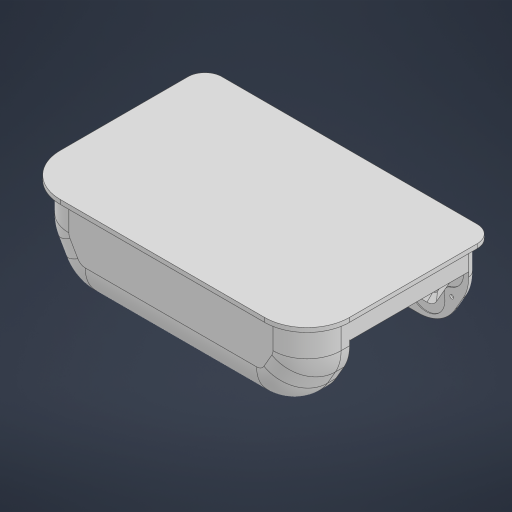
# Autodesk Inventor part: cap
Saved by Autodesk Inventor 2024 (Build 280153000, 153)
## iProperties
Created: 2024-05-06
Part Number: cap
Material: Generic
Document SubType Name: Modeling
Designer: markm
Density: 1 g/cm^3
Appearance: Default
Author: markm
Autodesk Inventor part; units mm, degrees
ref_plane "YZ Plane" through (0, 0, 0) normal (1, 0, 0) x (0, 1, 0)
ref_plane "XZ Plane" through (0, 0, 0) normal (0, 1, 0) x (-1, 0, 0)
ref_plane "XY Plane" through (0, 0, 0) normal (0, 0, 1) x (1, 0, 0)
sketch "Sketch18" plane through (0, 0, 0) normal (0, 1, 0) x (-1, 0, 0)
  line L0 (0, 55) -> (0, -55)
  line L1 (0, -55) -> (-85, -55)
  line L2 (-85, -55) -> (-85, 55)
  line L3 (0, 55) -> (-85, 55)
  point P0 (0, 0)
  point P1 (0, 0)
  dimension "d157" = 85
  dimension "d178" = 110
  constraints: 8 end point, 2 perpendicular, 1 coincident, 1 horizontal, 1 midpoint, 1 vertical
  measures "d157" distance between parallel lines of L2 L0
  measures "d178" distance between parallel lines of L3 L1
extrude "Extrusion22" add sketch "Sketch18" along normal blind 2.5
sketch "Sketch19" plane through (0, 0, 0) normal (0, -1, 0) x (1, 0, 0)
  line L0 (85, 55) -> (85, -55) projected
  line L1 (0, 55) -> (85, 55) projected
  line L2 (0, -55) -> (0, 55) projected
  line L3 (85, -55) -> (0, -55) projected
  line L4 (5, 50) -> (0, 50)
  line L5 (5, -50) -> (0, -50)
  line L6 (5, -50) -> (5, 50)
  line L7 (5, 50) -> (80, 50)
  line L8 (80, 50) -> (80, -50)
  line L9 (80, -50) -> (5, -50)
  point P0 (0, 0)
  dimension "d179" = 5
  constraints: 12 end point, 2 perpendicular, 2 point on line, 3 other
  measures "d179" distance between parallel lines of L3 L9
extrude "Extrusion23" add sketch "Sketch19" along normal blind 5 contours L4 L6 L5 L2 | L7 L8 L9 L6
sketch "Sketch20" plane through (0, -5, 0) normal (0, -1, 0) x (1, 0, 0)
  line L0 (0, 50) -> (0, -50) projected
  line L1 (80, 30) -> (0, 30)
  line L2 (80, -45) -> (0, -45)
  line L3 (80, 25) -> (0, 25)
  line L4 (0, -50) -> (80, -50) projected
  line L5 (80, -50) -> (80, 50) projected
  line L6 (80, 50) -> (0, 50) projected
  point P0 (0, 0)
  point P1 (0, 25)
  dimension "d167" = 5
  constraints: 6 end point, 3 perpendicular, 3 point on line, 1 parallel
  measures "d167" distance between parallel lines of L1 L3
extrude "Extrusion24" add sketch "Sketch20" along normal blind 45 contours L6 L5 L1 L0 | L1 L5 L3 L0 | L2 L5 L4 L0
sketch "Sketch21" plane through (0, 0, 0) normal (0, 0, 1) x (1, 0, 0)
  line L0 (0, -5) -> (80, -5)
  line L1 (0, -5) -> (0, -50)
  line L2 (80, -50) -> (0, -50)
  line L3 (80, -5) -> (80, -50)
  arc A0 (55, -47) -> (64.526279, -41.5) centre (55, -36) ccw construction
  line L4 (55, -36) -> (66, -16.947441) construction
  line L5 (0, -47) -> (55, -47) construction
  line L6 (64.526279, -41.5) -> (75.526279, -22.447441) construction
  arc A1 (75.526279, -22.447441) -> (74.887436, -10.465661) centre (66, -16.947441) ccw construction
  arc A2 (78.124356, -23.947441) -> (80, -16.947441) centre (66, -16.947441) ccw
  line L7 (78.124356, -23.947441) -> (67.124356, -43)
  arc A3 (55, -50) -> (67.124356, -43) centre (55, -36) ccw
  line L8 (55, -50) -> (0, -50)
  arc A4 (76.650635, -29.447441) -> (80, -16.947441) centre (55, -16.947441) ccw
  line L9 (76.650635, -29.447441) -> (64.78461, -50)
  arc A5 (50.350853, -50) -> (72.001488, -37.5) centre (50.350853, -25) ccw
  point P0 (0, 0)
  point P1 (55, -50)
  point P2 (50.350853, -50)
  dimension "d170" = 22
  dimension "d171" = 55
  dimension "d172" = 60
  dimension "d174" = 3
  dimension "d175" = 3
  dimension "d242" = 25
  constraints: 12 end point, 12 point on circle, 7 tangent, 6 centre point, 5 point on line, 2 equal radius, 2 parallel, 1 coincident, 3 other
  measures "d170" diameter of A0
  measures "d171" distance from line of L1 L4.start
  measures "d172" angle of L2 L4
  measures "d174" distance between parallel lines of L2 L5
  measures "d175" distance between parallel lines of L6 L7
  measures "d242" radius of A4
extrude "Extrusion25" cut sketch "Sketch21" along normal through all both and the other way through all contours L3 L2 L9 A4 | A5 A3 L2 | A3 A5 L9 L2
fillet "Fillet6" radius 20 1 edges at (80, -8.4737, 50)
fillet "Fillet6" radius 5 2 edges at (25.1754, -50, -50) (80, -8.4737, -50)
fillet "Fillet6" radius 25 1 edges at (85, 1.25, 55)
fillet "Fillet6" radius 10 1 edges at (85, 1.25, -55)
chamfer "Chamfer8" distance 5 distance2 2.5 5 edges at (74.1422, 0, 44.1422) (30, 0, 50) (80, 0, -7.5) (78.5356, 0, -48.5356) (37.5, 0, -50) measured on face at (80.5, 0, -7.5) measured on face at (37.5, 0, -50.5) measured on face at (78.8891, 0, -48.8891) measured on face at (74.4957, 0, 44.4957) measured on face at (30, 0, 50.5)
sketch "Sketch24" plane through (0, 2.5, -55) normal (-1, 0, 0) x (0, 0, 1)
  line L0 (110, -2.5) -> (105, -5) construction
  circle A0 centre (107.5, -3.75) radius 1
  point P0 (55, -2.5)
  dimension "d194" = 2
  constraints: 1 centre point, 1 midpoint
  measures "d194" diameter of A0
sketch3d "3D Sketch4"
  line L0 (0, -2.5, 50) -> (60, -2.5, 50)
  arc A0 (60, -2.5, 50) -> (80, -2.5, 30) centre (60, -2.5, 30) ccw
  line L1 (80, -2.5, 30) -> (80, -2.5, -45)
  arc A1 (80, -2.5, -45) -> (75, -2.5, -50) centre (75, -2.5, -45) ccw
  line L2 (75, -2.5, -50) -> (0, -2.5, -50)
sweep "Sweep4" cut profiles "Sketch24" path "3D Sketch4"
mirror "Mirror4" about plane through (0, 0, 0) normal (1, 0, 0)
ref_plane "Work Plane1" through (80, -16.947441, -10) normal (0, 0, 1) x (1, 0, 0)
sketch "Sketch26" plane through (80, -16.947441, -10) normal (0, 0, 1) x (1, 0, 0)
  line L0 (0, 11.947441) -> (0, 0)
  line L1 (-160, 11.947441) -> (0, 11.947441)
  line L2 (-160, 11.947441) -> (-160, 0)
  line L3 (-29.649147, -33.052559) -> (-130.350853, -33.052559)
  circle A0 centre (-25, -19.052559) radius 11
  circle A1 centre (-14.000001, 0) radius 11
  circle A2 centre (-146, 0) radius 11
  circle A3 centre (-47, -19.052559) radius 11
  circle A4 centre (-36.000001, 0) radius 11
  circle A5 centre (-69, -19.052559) radius 11
  circle A6 centre (-58.000001, 0) radius 11
  circle A7 centre (-91, -19.052559) radius 11
  circle A8 centre (-80.000001, 0) radius 11
  circle A9 centre (-113, -19.052559) radius 11
  circle A10 centre (-102.000001, 0) radius 11
  circle A11 centre (-135, -19.052559) radius 11
  circle A12 centre (-124.000001, 0) radius 11
  arc A13 (0, 0) -> (-14, 14) centre (-14, 0) ccw
  line L4 (-14, 14) -> (-146, 14)
  arc A14 (-146, 14) -> (-160, 0) centre (-146, 0) ccw
  arc A15 (-140.629165, -22.302559) -> (-135, -25.552559) centre (-135, -19.052559) ccw
  line L5 (-140.629165, -22.302559) -> (-151.629165, -3.25)
  arc A16 (-152.5, 0) -> (-151.629165, -3.25) centre (-146, 0) ccw
  line L6 (-152.5, 0) -> (-152.5, 4.447441)
  line L7 (-152.5, 4.447441) -> (-7.5, 4.447441)
  line L8 (-7.5, 4.447441) -> (-7.5, 0)
  arc A17 (-8.370835, -3.25) -> (-7.5, 0) centre (-14.000001, 0) ccw
  line L9 (-8.370835, -3.25) -> (-19.370835, -22.302559)
  arc A18 (-25, -25.552559) -> (-19.370835, -22.302559) centre (-25, -19.052559) ccw
  line L10 (-25, -25.552559) -> (-135, -25.552559)
  arc A19 (-146, 6.5) -> (-152.5, 0) centre (-146, 0) ccw
  line L11 (-146, 6.5) -> (-14, 6.5)
  arc A20 (-7.5, 0) -> (-14, 6.5) centre (-14, 0) ccw
  arc A21 (-3.349365, -12.5) -> (0, 0) centre (-25, 0) ccw
  arc A22 (-160, 0) -> (-156.650635, -12.5) centre (-135, 0) ccw
  line L12 (-152.001488, -20.552559) -> (-156.650635, -12.5)
  line L13 (-7.998512, -20.552559) -> (-3.349365, -12.5)
  arc A23 (-152.001488, -20.552559) -> (-130.350853, -33.052559) centre (-130.350853, -8.052559) ccw
  arc A24 (-29.649147, -33.052559) -> (-7.998512, -20.552559) centre (-29.649147, -8.052559) ccw
  point P0 (-80, 16.947441)
  point P1 (-153.297852, 11.947441)
  point P2 (-6.702148, 11.947441)
  point P3 (-7.5, 0)
  point P4 (-135, 0.003127)
  point P5 (-140.5, -9.526279)
  point P6 (-124, -19.052559)
  point P7 (-102, -19.052559)
  point P8 (-80, -19.052559)
  point P9 (-58, -19.052559)
  point P10 (-36, -19.052559)
  point P11 (-19.498599, -9.527088)
  point P12 (-25.000001, 0)
  point P13 (-47.000001, 0)
  point P14 (-69.000001, 0)
  point P15 (-91.000001, 0)
  point P16 (-113.000001, 0)
  dimension "d205" = 22
  dimension "d208" = 22
  dimension "d213" = 7.5
  constraints: 21 centre point, 16 end point, 16 point on circle, 3 coincident, 3 equal radius, 2 horizontal, 1 tangent, 24 other
  measures "d205" diameter of A0
  measures "d208" distance of A0.centre A3.centre
  measures "d213" distance between parallel lines of L3 L10
extrude "Extrusion28" add sketch "Sketch26" against normal up to surface (35 mm away) contours L0 A13 L1 | A14 L2 L1
extrude "Extrusion29" cut sketch "Sketch26" against normal up to surface (35 mm away) contours L1 A14 L4 A13
extrude "Extrusion31" cut sketch "Sketch26" against normal blind 35.5 contours A0 L10 A18 L9 | L9 A18 L10 A0 | A0 A4 A1 | A1 L7 A20 A17 L9 | L9 A17 L8 L7 A20 L11 A1 | A3 A4 A0 | A3 L10 | A3 L10 | A4 L7 | A3 A6 A4 | A1 L11 A20 L7 | L7 A4 L11 | A20 L7 L8 | A3 A5 A6 | A6 L7 | A5 L10 | A5 L10 | L11 A4 | A5 A8 A6 | L7 A6 L11 | A5 A7 A8 | A8 L7 | L11 A6 | A7 L10 | A7 L10 | A7 A10 A8 | L7 A8 L11 | A7 A9 A10 | A10 L7 | L11 A8 | A9 L10 | A9 L10 | A9 A12 A10 | L7 A10 L11 | A9 A11 A12 | A12 L7 | L11 A10 | A11 L10 A15 L5 | A11 L5 A15 L10 | A11 A2 A12 | L7 A12 L11 | A2 L5 A16 A19 L7 | L11 A12 | A2 L11 A19 L7 L6 A16 L5 | L7 A19 L11 A2 | A19 L6 L7
fillet "Fillet9" radius 5 13 edges at (-60.5, -26.4737, -45.25) (-44, -36, -45.25) (-22, -36, -45.25) (44, -36, -45.25) (0, -36, -45.25) (22, -36, -45.25) (-55, -16.9443, -45.25) (33, -16.9474, -45.25) (55, -16.9474, -45.25) (11, -16.9474, -45.25) (-33, -16.9474, -45.25) (-11, -16.9474, -45.25) (60.5014, -26.4745, -45.25)
extrude "Extrusion30" cut sketch "Sketch26" against normal blind 39 contours L9 A18 L10 A0 | A0 A1 L9 | L10 A3 A0 | A0 A4 A1 | A1 L7 A20 A17 L9 | A3 A4 A0 | A3 L10 | A4 L7 | A4 L7 A1 | A3 A6 A4 | L10 A5 A3 | L7 A4 L11 A1 | A1 L11 A20 L7 | L7 A4 L11 | A3 A5 A6 | A6 L7 | A6 L7 A4 | A5 L10 | L7 A6 L11 A4 | A5 A8 A6 | L7 A6 L11 | L10 A7 A5 | A5 A7 A8 | A8 L7 | A8 L7 A6 | L7 A8 L11 A6 | A7 L10 | A7 A10 A8 | L7 A8 L11 | L10 A9 A7 | A7 A9 A10 | A10 L7 | A10 L7 A8 | L7 A10 L11 A8 | A9 L10 | A9 A12 A10 | L7 A10 L11 | L10 A11 A9 | A9 A11 A12 | A12 L7 | A12 L7 A10 | L7 A12 L11 A10 | A11 L10 A15 L5 | A11 A2 A12 | L7 A12 L11 | L5 A2 A11 | A2 L5 A16 A19 L7 | A2 L7 A12 | L7 A2 L11 A12 | L7 A19 L11 A2 picked at (-24.956945, -19.127133) picked at (-44.033604, -18.431276) picked at (-72.50543, -19.057181) picked at (-94.50543, -19.057181) picked at (-116.50543, -19.057181) picked at (-135.043055, -19.127132)
chamfer "Chamfer10" distance 3.5 angle 45 10 edges at (58.25, -41.6292, -49) (0, -42.5, -49) (-58.25, -41.6292, -49) (-66.1292, -29.7237, -49) (-70.5962, -12.3512, -49) (-72.2785, -18.6298, -49) (0, -10.4474, -49) (72.2785, -18.6298, -49) (70.5962, -12.3512, -49) (66.1292, -29.7237, -49)
sketch "Sketch27" plane through (75, -16.947441, -50) normal (0, 0, -1) x (-1, 0, 0)
  line L0 (0, 14.447441) -> (150, 14.447441) construction
  line L1 (0, 0) -> (0, 14.447441) construction
  line L2 (125.350853, -28.052559) -> (24.649147, -28.052559) construction
  line L3 (150, 0) -> (150, 14.447441) construction
  arc A0 (9.300915, -16.497256) -> (5.863415, -10.543331) centre (4.437694, -15.335754) ccw construction
  arc A1 (9.300915, -16.497256) -> (27.5625, -27.040587) centre (20, -19.052559) ccw construction
  arc A2 (34.4375, -27.040587) -> (27.5625, -27.040587) centre (31, -30.671509) ccw construction
  arc A3 (34.4375, -27.040587) -> (49.5625, -27.040587) centre (42, -19.052559) ccw construction
  arc A4 (56.4375, -27.040587) -> (49.5625, -27.040587) centre (53, -30.671509) ccw construction
  arc A5 (56.4375, -27.040587) -> (71.5625, -27.040587) centre (64, -19.052559) ccw construction
  arc A6 (78.4375, -27.040587) -> (71.5625, -27.040587) centre (75, -30.671509) ccw construction
  arc A7 (78.4375, -27.040587) -> (93.5625, -27.040587) centre (86, -19.052559) ccw construction
  arc A8 (100.4375, -27.040587) -> (93.5625, -27.040587) centre (97, -30.671509) ccw construction
  arc A9 (100.4375, -27.040587) -> (115.5625, -27.040587) centre (108, -19.052559) ccw construction
  arc A10 (122.4375, -27.040587) -> (115.5625, -27.040587) centre (119, -30.671509) ccw construction
  arc A11 (122.4375, -27.040587) -> (140.699085, -16.497256) centre (130, -19.052559) ccw construction
  arc A12 (144.136585, -10.543331) -> (140.699085, -16.497256) centre (145.562306, -15.335754) ccw construction
  arc A13 (144.136585, -10.543331) -> (133.4375, 7.988029) centre (141, 0) ccw construction
  arc A14 (126.562501, 7.988029) -> (133.4375, 7.988029) centre (130.000001, 11.618951) ccw construction
  arc A15 (126.562501, 7.988029) -> (111.437501, 7.988028) centre (119.000001, 0) ccw construction
  arc A16 (104.562501, 7.988028) -> (111.437501, 7.988028) centre (108.000001, 11.61895) ccw construction
  arc A17 (104.562501, 7.988028) -> (89.437501, 7.988028) centre (97.000001, 0) ccw construction
  arc A18 (82.562501, 7.988028) -> (89.437501, 7.988028) centre (86.000001, 11.61895) ccw construction
  arc A19 (82.562501, 7.988028) -> (67.437501, 7.988028) centre (75.000001, 0) ccw construction
  arc A20 (60.562501, 7.988028) -> (67.437501, 7.988028) centre (64.000001, 11.61895) ccw construction
  arc A21 (60.562501, 7.988028) -> (45.437501, 7.988028) centre (53.000001, 0) ccw construction
  arc A22 (38.562501, 7.988028) -> (45.437501, 7.988028) centre (42.000001, 11.61895) ccw construction
  arc A23 (38.562501, 7.988028) -> (23.437501, 7.988028) centre (31.000001, 0) ccw construction
  arc A24 (16.562501, 7.988028) -> (23.437501, 7.988028) centre (20.000001, 11.61895) ccw construction
  arc A25 (16.562501, 7.988028) -> (5.863415, -10.543331) centre (9.000001, 0) ccw construction
  arc A26 (155, 0) -> (141, 14) centre (141, 0) ccw construction
  line L4 (24.649147, -33.052559) -> (125.350853, -33.052559) construction
  arc A27 (9, 14) -> (-5, 0) centre (9, 0) ccw construction
  line L5 (141, 14) -> (9, 14) construction
  line L6 (-0.526279, -5.5) -> (10.473721, -24.552559) construction
  arc A28 (10.473721, -24.552559) -> (20, -30.052559) centre (20, -19.052559) ccw construction
  line L7 (20, -30.052559) -> (130, -30.052559) construction
  arc A29 (130, -30.052559) -> (139.526279, -24.552559) centre (130, -19.052559) ccw construction
  line L8 (139.526279, -24.552559) -> (150.526279, -5.5) construction
  arc A30 (150.526279, -5.5) -> (152, 0) centre (141, 0) ccw construction
  arc A31 (152, 0) -> (141, 11) centre (141, 0) ccw construction
  line L9 (141, 11) -> (9, 11) construction
  arc A32 (9, 11) -> (-2, 0) centre (9, 0) ccw construction
  arc A33 (-2, 0) -> (-0.526279, -5.5) centre (9.000001, 0) ccw construction
  circle A34 centre (4.973721, -15.026279) radius 1.1
  circle A35 centre (4.973721, -15.026279) radius 2
  circle A36 centre (31, -30.052559) radius 1.1
  circle A37 centre (31, -30.052559) radius 2
  line L10 (31, -30.671509) -> (31, -30.052559) construction
  arc A38 (151.650635, -12.5) -> (155, 0) centre (130, 0) ccw
  line L11 (147.001488, -20.552559) -> (151.650635, -12.5)
  line L12 (2.998512, -20.552559) -> (-1.650635, -12.5)
  arc A39 (-5, 0) -> (-1.650635, -12.5) centre (20, 0) ccw
  arc A40 (0, 0) -> (2.679492, -10) centre (20, 0) ccw
  line L13 (7.328639, -18.052559) -> (2.679492, -10)
  line L14 (142.671361, -18.052559) -> (147.320508, -10)
  arc A41 (147.320508, -10) -> (150, 0) centre (130, 0) ccw
  arc A42 (125.350853, -33.052559) -> (147.001488, -20.552559) centre (125.350853, -8.052559) ccw
  arc A43 (2.998512, -20.552559) -> (24.649147, -33.052559) centre (24.649147, -8.052559) ccw
  arc A44 (7.328639, -18.052559) -> (24.649147, -28.052559) centre (24.649147, -8.052559) ccw
  arc A45 (125.350853, -28.052559) -> (142.671361, -18.052559) centre (125.350853, -8.052559) ccw
  point P0 (75, 16.947441)
  dimension "d229" = 2.2
  dimension "d230" = 4
  constraints: 12 point on circle, 10 centre point, 10 end point, 2 coincident, 2 equal radius, 1 midpoint, 1 tangent, 1 vertical, 2 other
  measures "d229" diameter of A34
  measures "d230" diameter of A35
extrude "Extrusion32" cut sketch "Sketch27" against normal blind 4 contours A34 L13 | A34 L13 A35 | L13 A34 | A34 L13 A35
extrude "Extrusion33" cut sketch "Sketch27" against normal up to next contours A34 L13 | L13 A34
extrude "Extrusion34" cut sketch "Sketch27" against normal blind 4 contours A36 | A37
extrude "Extrusion35" cut sketch "Sketch27" against normal up to next contours A36
mirror "Mirror6" about plane through (0, 0, 0) normal (1, 0, 0) of "Extrusion32", "Extrusion33"
pattern_linear "Rectangular Pattern3" count 5 spacing 22 along (-1, 0, 0) of "Extrusion34", "Extrusion35"
mirror "Mirror5" about plane through (80, -16.947441, -10) normal (0, 0, 1) of "Extrusion30", "Extrusion29", "Extrusion28", "Extrusion31", "Fillet9", "Chamfer10", "Extrusion32", "Extrusion33", "Extrusion34", "Extrusion35", "Mirror6", "Rectangular Pattern3"
thicken "Thicken2" operation cut thickness 0.25 both sides no extend neighbours no toward (0.9907219, 0.135905, 0) faces at (79.870106, -15.044771, -10) (22, -2.947441, 13.333333) (-73.398382, -5.06199, -21.666667)
body "Solid4"
